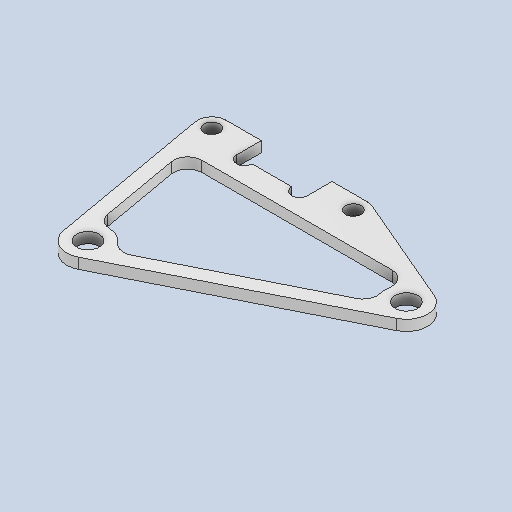
# Autodesk Inventor part: momo
Saved by Autodesk Inventor 2025.1 (Build 291241000, 241)
## iProperties
Created: 2024-09-02
Part Number: momo
Material: アルミニウム 2014-T4
Document SubType Name: Modeling
Designer: right
Density: 2.8 g/cm^3
Appearance: サテン
Mass: 1.2091 g
Surface Area: 9.27253 cm^2
Volume: 0.431823 cm^3
Author: right
Autodesk Inventor part; units mm, degrees
ref_plane "YZ Plane" through (0, 0, 0) normal (1, 0, 0) x (0, 1, 0)
ref_plane "XZ Plane" through (0, 0, 0) normal (0, 1, 0) x (-1, 0, 0)
ref_plane "XY Plane" through (0, 0, 0) normal (0, 0, 1) x (1, 0, 0)
sketch "スケッチ1" plane through (0, 0, 0) normal (0, 1, 0) x (-1, 0, 0)
  line L0 (5, 0) -> (-5, 0)
  line L1 (-5, 0) -> (-5, -3)
  line L2 (-5, -3) -> (5, -3)
  line L3 (5, -3) -> (5, 0)
  circle A0 centre (3.9, 0) radius 1.1
  line L4 (0, -3) -> (0, 0) construction
  circle A1 centre (-3.9, 0) radius 1.1
  line L5 (-5, -1.5) -> (5, -1.5) construction
  circle A2 centre (3.9, -3) radius 1.1
  circle A3 centre (-3.9, -3) radius 1.1
  circle A4 centre (-10, -1.5) radius 1.1
  circle A5 centre (10, -1.5) radius 1.1
  circle A6 centre (10, -1.5) radius 2
  circle A7 centre (-10, -1.5) radius 2
  line L6 (10, -3.5) -> (-10, -3.5)
  line L7 (-5, -3) -> (-5, -3.5)
  line L8 (5, -3) -> (5, -3.5)
  circle A8 centre (-25, 6) radius 1.6
  circle A9 centre (5, 21) radius 1.6
  line L9 (-25, 6) -> (5, 6) construction
  line L10 (5, 6) -> (5, 21) construction
  line L11 (5, 21) -> (-25, 6) construction
  circle A10 centre (-25, 6) radius 3
  circle A11 centre (5, 21) radius 3
  line L12 (11.9694, -1.1513) -> (7.954, 21.5231)
  line L13 (-10.7862, -3.339) -> (-26.1793, 3.2415)
  line L14 (-26.3416, 8.6833) -> (3.6584, 23.6833)
  point P0 (-2.8, 0)
  point P1 (2.8, 0)
  dimension "d2" = 2.2
  dimension "d0" = 10
  dimension "d1" = 3
  dimension "d3" = 2.2
  dimension "d4" = 5
  dimension "d5" = 4
  dimension "d6" = 4
  dimension "d7" = 3.2
  dimension "d8" = 3.2
  dimension "d9" = 15
  dimension "d10" = 30
  dimension "d11" = 6
  dimension "d12" = 6
  dimension "d15" = 15
  dimension "d17" = 6
  constraints: 30 end point, 11 centre point, 8 point on circle, 8 tangent, 5 perpendicular, 4 coincident, 4 symmetric about line, 3 midpoint, 3 point on line, 2 horizontal, 2 horizontal alignment, 2 parallel, 1 vertical alignment, 7 other
  measures "d0" distance of L1.end L2.end
  measures "d1" distance between parallel lines of L0 L2
  measures "d3" diameter of A4
  measures "d4" distance from line of L1 A4.centre
  measures "d5" diameter of A6
  measures "d6" diameter of A7
  measures "d7" diameter of A8
  measures "d8" diameter of A9
  measures "d9" distance of L9.end L10.end
  measures "d10" distance of L9.start L9.end
  measures "d11" diameter of A10
  measures "d12" diameter of A11
  measures "d15" horizontal distance of A4.centre L9.start
  measures "d17" distance from line of L0 A10.centre
extrude "押し出し1" add sketch "スケッチ1" along normal blind 1.5 contours A1 L1 L7 L6 A7 L13 A10 L14 A11 L12 A6 L8 L3 A0 L0 | A7 | A6 | A10 | A11
sketch "スケッチ2" plane through (0, 1.5, 0) normal (0, 1, 0) x (1, 0, 0)
  line L0 (-9.1854, -3.1) -> (-5.7511, -22.4936)
  line L1 (-5.7511, -22.4936) -> (27.378, -5.929)
  line L2 (27.378, -5.929) -> (20.7603, -3.1)
  line L3 (20.7603, -3.1) -> (-9.1854, -3.1)
  line L4 (10, 3.5) -> (5, 3.5) projected
  line L5 (26.1793, -3.2415) -> (10.7862, 3.339) projected
  line L6 (-11.9694, 1.1513) -> (-7.954, -21.5231) projected
  line L7 (-3.6584, -23.6833) -> (26.3416, -8.6833) projected
  arc A0 (2.8, 0) -> (5, 0) centre (3.9, 0) ccw projected
  line L8 (-3.6584, -23.6833) -> (26.3416, -8.6833) projected
  arc A1 (26.3416, -8.6833) -> (26.1793, -3.2415) centre (25, -6) ccw projected
  line L9 (26.1793, -3.2415) -> (10.7862, 3.339) projected
  arc A2 (10.7862, 3.339) -> (10, 3.5) centre (10, 1.5) ccw projected
  line L10 (10, 3.5) -> (5, 3.5) projected
  line L11 (5, 3.5) -> (5, 0) projected
  arc A3 (2.8, 0) -> (5, 0) centre (3.9, 0) ccw projected
  line L12 (2.8, 0) -> (-2.8, 0) projected
  arc A4 (-5, 0) -> (-2.8, 0) centre (-3.9, 0) ccw projected
  line L13 (-5, 0) -> (-5, 3.5) projected
  line L14 (-5, 3.5) -> (-10, 3.5) projected
  arc A5 (-10, 3.5) -> (-11.9694, 1.1513) centre (-10, 1.5) ccw projected
  line L15 (-11.9694, 1.1513) -> (-7.954, -21.5231) projected
  arc A6 (-7.954, -21.5231) -> (-3.6584, -23.6833) centre (-5, -21) ccw projected
  circle A7 centre (10, 1.5) radius 1.1 projected
  circle A8 centre (25, -6) radius 1.6 projected
  circle A9 centre (-10, 1.5) radius 1.1 projected
  circle A10 centre (-5, -21) radius 1.6 projected
  circle A11 centre (-5, -21) radius 3
  circle A12 centre (25, -6) radius 3
  point P0 (0, 0)
  point P1 (3.9, -1.1)
  point P2 (-6.4779, -18.3893)
  point P3 (-2.023, -20.6295)
  point P4 (22.9174, -8.1593)
  point P5 (22.7923, -3.9687)
  dimension "d18" = 2
  dimension "d19" = 2
  dimension "d20" = 2
  dimension "d22" = 2
  constraints: 8 end point, 4 parallel, 2 coincident, 1 centre point, 1 concentric, 1 point on circle, 3 other
  measures "d18" distance between parallel lines of L5 L2
  measures "d19" distance between parallel lines of L7 L1
  measures "d20" distance between parallel lines of L6 L0
  measures "d22" distance from line of point (3.9, -1.1) L3
extrude "押し出し2" cut sketch "スケッチ2" against normal through all contours L3 L2 A12 L1 A11 L0
fillet "フィレット1" radius 2 6 edges at (22.7923, 0.75, 3.9687) (22.9174, 0.75, 8.1593) (20.7603, 0.75, 3.1) (-9.1854, 0.75, 3.1) (-2.023, 0.75, 20.6295) (-6.4779, 0.75, 18.3893)
equation "\"d18\" = d22"
equation "\"d19\" = d18"
equation "\"d20\" = d19"
